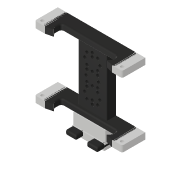
# Autodesk Inventor part: e4-phone_1piece pivot
Saved by Autodesk Inventor 2018 (Build 220112000, 112)
## iProperties
Created: 2019-01-02
Part Number: e4-phone_1piece pivot
Material: Generic
Document SubType Name: Modeling
Designer: ball
Density: 1 g/cm^3
Appearance: Default
Author: ball
Autodesk Inventor part; units mm, degrees
ref_plane "YZ Plane" through (0, 0, 0) normal (1, 0, 0) x (0, 1, 0)
ref_plane "XZ Plane" through (0, 0, 0) normal (0, 1, 0) x (-1, 0, 0)
ref_plane "XY Plane" through (0, 0, 0) normal (0, 0, 1) x (1, 0, 0)
ref_plane "Work Plane1" through (-89.882, 196577.8405, 29.6599) normal (0, 0, -1) x (-1, 0, 0)
sketch "Sketch3" plane through (0, -8, 26.5711) normal (1, 0, 0) x (0, 1, 0)
  line L0 (30.2, 3.0888) -> (-125.2, 3.0888) construction
  line L1 (-75, -26.5711) -> (0, -26.5711) construction
  line L2 (8, -26.5711) -> (0, -26.5711)
  line L3 (0, -26.5711) -> (0, 3.0888)
  line L4 (0, 3.0888) -> (8, 3.0888)
  line L5 (8, 3.0888) -> (8, -26.5711)
  line L6 (-83, 0) -> (-83, -23.5711) construction
  line L7 (-83, -26.5711) -> (-75, -26.5711)
  line L8 (-75, -26.5711) -> (-75, 3.0888)
  line L9 (-75, 3.0888) -> (-83, 3.0888)
  line L10 (-83, 3.0888) -> (-83, -26.5711)
  constraints: 16 end point, 4 parallel, 2 horizontal, 2 perpendicular, 2 point on line
extrude "Extrusion2" add sketch "Sketch3" along normal blind 10 and the other way blind 3
sketch "Sketch4" plane through (-3, 0, 29.6599) normal (0, 1, 0) x (1, 0, 0)
  circle A0 centre (8, 5) radius 1.965
  line L0 (13, 29.6599) -> (13, 0) projected
  line L1 (-109.6757, 0) -> (33.4459, 0) projected
  point P0 (3, 29.6599)
  dimension "d19" = 3.93
  dimension "d20" = 5
  dimension "d21" = 5
  constraints: 1 centre point
  measures "d19" diameter of A0
  measures "d20" distance from line of L0 A0.centre
  measures "d21" distance from line of L1 A0.centre
hole "Hole2" at (5, 0, 24.6599) direction (0, -1, 0) diameter 3.93 end through all
fillet "Fillet1" radius 2 2 edges at (10, -4, 29.6599) (10, -87, 29.6599)
sketch "Sketch5" plane through (-92.2297, -8, 3) normal (-1, 0, 0) x (0, -1, 0)
  line L0 (-8, -3) -> (0, -3) projected
  line L1 (0, -3) -> (0, 26.6599) projected
  line L2 (-8, -3) -> (0, -3)
  line L3 (0, -3) -> (0, 26.6599)
  line L4 (0, 26.6599) -> (-8, 26.6599)
  line L5 (-8, 26.6599) -> (-8, -3)
  line L6 (83, -3) -> (75, -3) projected
  line L7 (83, 26.6599) -> (75, 26.6599) projected
  line L8 (83, -3) -> (75, -3)
  line L9 (75, -3) -> (75, 26.6599)
  line L10 (75, 26.6599) -> (83, 26.6599)
  line L11 (83, 26.6599) -> (83, -3)
  constraints: 16 end point, 4 parallel, 2 horizontal, 2 perpendicular
extrude "Extrusion3" add sketch "Sketch5" along normal blind 10 and the other way blind 3
sketch "Sketch6" plane through (-102.2297, 0, 0) normal (0, 1, 0) x (1, 0, 0)
  circle A0 centre (5, -24.6599) radius 1.965
  line L0 (0, -29.6599) -> (0, 0) projected
  line L1 (13, -29.6599) -> (0, -29.6599) projected
  point P0 (102.2297, 0)
  dimension "d34" = 3.93
  dimension "d35" = 5
  dimension "d36" = 5
  constraints: 1 centre point
  measures "d34" diameter of A0
  measures "d35" distance from line of L0 A0.centre
  measures "d36" distance from line of L1 A0.centre
hole "Hole3" at (-97.2297, 0, 24.6599) direction (0, -1, 0) diameter 3.93 end through all
fillet "Fillet2" radius 2 2 edges at (-102.2297, -4, 29.6599) (-102.2297, -87, 29.6599)
sketch "Sketch9" plane through (-27.41, -83, 0) normal (0, 0, -1) x (-1, 0, 0)
  line L0 (-24.41, -8) -> (61.8197, -8) construction
  line L1 (-1.9451, -8) -> (-1.9451, -26) construction
  line L2 (39.3549, -26) -> (39.3549, -8) construction
  line L3 (0.0549, -28) -> (37.3549, -28) construction
  line L4 (-1.9451, -8) -> (39.3549, -8)
  line L5 (39.3549, -8) -> (39.3549, -30)
  line L6 (-1.9451, -30) -> (-1.9451, -8)
  line L7 (-1.9451, -30) -> (39.3549, -30)
  point P0 (-27.41, 83)
  dimension "d50" = 2
  constraints: 8 end point, 2 parallel, 1 horizontal, 1 perpendicular
  measures "d50" distance between parallel lines of L3 L7
extrude "Extrusion5" add sketch "Sketch9" against normal blind 17.12
sketch "Sketch12" plane through (-27.41, -83, 17.12) normal (0, 0, 1) x (1, 0, 0)
  line L0 (1.9451, -8) -> (-39.3549, -8) construction
  line L1 (1.9451, -30) -> (1.9451, -8) construction
  line L2 (1.9451, -21.9992) -> (-39.4839, -21.9992) construction
  line L3 (-39.3549, -8) -> (-39.3549, -30) projected
  line L4 (-39.3549, -8) -> (1.9451, -8)
  line L5 (1.9451, -8) -> (1.9451, -21.9992)
  line L6 (1.9451, -21.9992) -> (-39.3549, -21.9992)
  line L7 (-39.3549, -21.9992) -> (-39.3549, -8)
  point P0 (27.41, 83)
  constraints: 10 end point, 2 parallel, 2 perpendicular, 1 horizontal, 1 point on line
extrude "Extrusion6" cut sketch "Sketch12" against normal blind 1.524
body "Solid2"
